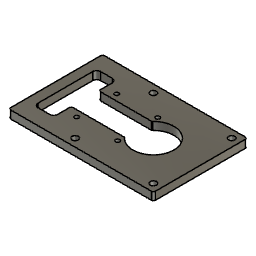
headcamera_plate_3 (Autodesk Fusion 360 design; units mm, degrees)
Autodesk Fusion 360 part; units mm, degrees
note: some values were not read from the file. Set by a fixed rule: the direction of a hole.
sketch "スケッチ1" plane through (0, 0, 0) normal (0, 0, 1) x (1, 0, 0)
  circle A0 centre (0, 0) radius 10.5
  line L0 (-50, 24) -> (24, 24)
  line L1 (24, 24) -> (24, -24)
  line L2 (24, -24) -> (-50, -24)
  line L3 (-50, -24) -> (-50, 24)
  line L4 (-29, 10.25) -> (-8, 10.25)
  line L5 (-8, 10.25) -> (-8, -10.25)
  line L6 (-8, -10.25) -> (-29, -10.25)
  line L7 (-29, -10.25) -> (-29, 10.25)
  line L8 (-20, 20) -> (20, 20)
  line L9 (20, 20) -> (20, -20)
  line L10 (20, -20) -> (-20, -20)
  line L11 (-20, -20) -> (-20, 20)
  line L12 (-45, 16) -> (-35, 16)
  line L13 (-35, 16) -> (-35, -16)
  line L14 (-35, -16) -> (-45, -16)
  line L15 (-45, -16) -> (-45, 16)
  line L16 (-35, 7) -> (0, 7)
  line L17 (0, 7) -> (0, -7)
  line L18 (0, -7) -> (-35, -7)
  line L19 (-35, -7) -> (-35, 7)
  point P0 (24, 0)
  point P1 (-8, 0)
  point P2 (0, 20)
  point P3 (20, 0)
  point P4 (-35, 0)
  dimension "d1" = 21
  dimension "d2" = 48
  dimension "d3" = 24
  dimension "d4" = 50
  dimension "d5" = 8
  dimension "d6" = 21
  dimension "d7" = 20.5
  dimension "d13" = 40
  dimension "d14" = 40
  dimension "d15" = 32
  dimension "d16" = 10
  dimension "d17" = 5
  dimension "d21" = 14
  constraint coincident A0.centre origin
  constraint horizontal L0
  constraint vertical L1
  constraint horizontal L2
  constraint vertical L3
  constraint midpoint L1 P0
  constraint horizontal A0.centre P0
  constraint horizontal L4
  constraint vertical L5
  constraint horizontal L6
  constraint vertical L7
  constraint midpoint L5 P1
  constraint horizontal A0.centre P1
  constraint horizontal L8
  constraint vertical L9
  constraint horizontal L10
  constraint vertical L11
  constraint midpoint L8 P2
  constraint midpoint L9 P3
  constraint horizontal A0.centre P3
  constraint vertical A0.centre P2
  constraint horizontal L12
  constraint vertical L13
  constraint horizontal L14
  constraint vertical L15
  constraint coincident L13 P4
  constraint midpoint L13 P4
  constraint horizontal A0.centre P4
  constraint horizontal L16
  constraint vertical L17
  constraint horizontal L18
  constraint vertical L19
  constraint coincident P4 L19
  constraint midpoint A0.centre L17
  measures "d1" diameter of A0
  measures "d2" distance of L0.end L1.end
  measures "d3" distance of A0.centre L1
  measures "d4" distance of A0.centre L3
  measures "d5" distance of A0.centre L5
  measures "d6" distance of L4.start L4.end
  measures "d7" distance of L4.start L6.end
  measures "d13" distance of L8.start L8.end
  measures "d14" distance of L8.end L9.end
  measures "d15" distance of L12.start L14.end
  measures "d16" distance of L12.start L12.end
  measures "d17" distance of L3 L15
  measures "d21" distance of L16 L18
extrude "押し出し1" add sketch "スケッチ1" along normal blind 4 contours A0 L4 L5 L6 L8 L9 L10 L11 L16 L18 | A0 L5 L16 | A0 L5 L18 | L4 L5 L11 L16 | L5 L6 L11 L18 | L4 L7 L11 L16 | L6 L7 L11 L18 | L0 L1 L2 L3
hole "穴1" at (-8, -10.25, 0) at (-29, -10.25, 0) at (-29, 10.25, 0) at (-8, 10.25, 0) direction (0, 0, 1) diameter 2.1 depth 17 tip angle 118
hole "穴2" at (-20, 20, 0) at (20, 20, 0) at (20, -20, 0) at (-20, -20, 0) direction (0, 0, 1) diameter 3.2 depth 10 tip angle 118
fillet "フィレット1" radius 1 8 edges at (-50, -24, 2) (24, -24, 2) (-50, 24, 2) (24, 24, 2) (-8, 6.8007, 2) (-8, -7, 2) (-35, 7, 2) (-35, -7, 2)
fillet "フィレット2" radius 2 4 edges at (-45, 16, 2) (-45, -16, 2) (-35, -16, 2) (-35, 16, 2)
